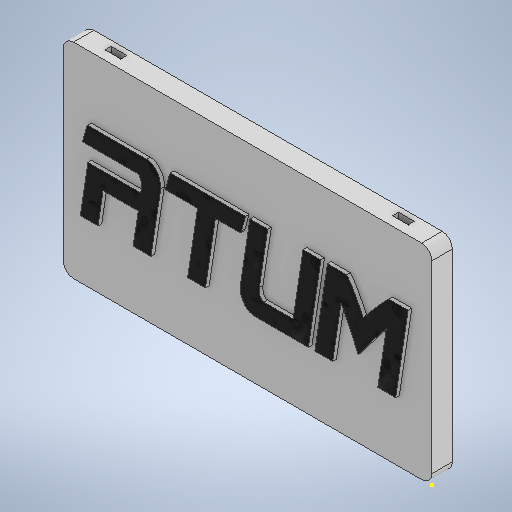
# Autodesk Inventor part: custom plate
Saved by Autodesk Inventor 2025.2 (Build 292293000, 293)
## iProperties
Created: 2024-12-05
Part Number: custom plate
Material: Generic
Document SubType Name: Modeling
Designer: Hunter Mathis
Density: 1 g/cm^3
Appearance: Default
Author: Hunter Mathis
Autodesk Inventor part; units mm, degrees
ref_plane "YZ Plane" through (0, 0, 0) normal (1, 0, 0) x (0, 1, 0)
ref_plane "XZ Plane" through (0, 0, 0) normal (0, 1, 0) x (-1, 0, 0)
ref_plane "XY Plane" through (0, 0, 0) normal (0, 0, 1) x (1, 0, 0)
sketch "Sketch1" plane through (0, 0, 0) normal (0, 0, 1) x (1, 0, 0)
  line L0 (0, 0) -> (-114.3, 0)
  line L1 (-114.3, 0) -> (-114.3, 63.5)
  line L2 (-114.3, 63.5) -> (0, 63.5)
  line L3 (0, 63.5) -> (0, 0)
  dimension "d7" = 114.3
  dimension "d8" = 63.5
  constraints: 8 end point, 2 parallel, 1 horizontal, 1 perpendicular
  measures "d7" distance of L1.end L2.end
  measures "d8" distance of L0.end L1.end
extrude "Extrusion1" add sketch "Sketch1" along normal blind 6.35
sketch "Sketch2" plane through (0, 0, 6.35) normal (0, 0, 1) x (1, 0, 0)
  line L0 (0, 0) -> (0, 63.5) projected
  line L1 (-114.3, 63.5) -> (-114.3, 0) projected
  line L2 (-114.3, 0) -> (0, 0) projected
  line L3 (0, 63.5) -> (-114.3, 63.5) projected
sketch "Sketch3" plane through (0, 0, 6.35) normal (0, 0, 1) x (1, 0, 0)
  line L0 (-110.6716, 35.2666) -> (-52.0005, 35.2666) construction
  line L1 (-52.0005, 35.2666) -> (-52.0005, 28.3217) construction
  line L2 (-52.0005, 28.3217) -> (-110.6716, 28.3217) construction
  line L3 (-110.6716, 28.3217) -> (-110.6716, 35.2666) construction
  line L4 (-114.3, 63.5) -> (-114.3, 0) projected
  line L5 (-107.8928, 19.0941) -> (-105.5257, 34.5523)
  line L6 (-105.5257, 34.5523) -> (-89.1412, 34.5523)
  line L7 (-89.1412, 34.5523) -> (-88.8942, 36.0343)
  spline S0 degree 2 poles (-88.8942, 36.0343) (-88.8119, 36.693) (-88.9766, 37.8663) (-89.3882, 38.7514) (-89.9852, 39.2659) (-90.3145, 39.2659) knots 0 0 0 1 2 3 4 4 4
  line L8 (-90.3145, 39.2659) -> (-107.1929, 39.2659)
  spline S1 degree 2 poles (-107.1929, 39.2659) (-106.9048, 40.3157) (-106.2667, 42.8063) (-105.9168, 43.8561) knots 0 0 0 1 2 2 2
  line L9 (-105.9168, 43.8561) -> (-105.6492, 44.4941)
  line L10 (-105.6492, 44.4941) -> (-87.3505, 44.4941)
  spline S2 degree 2 poles (-87.3505, 44.4941) (-86.6301, 44.4941) (-85.0451, 43.7737) (-83.7484, 42.3123) (-82.925, 40.1922) (-82.9662, 38.7308) knots 0 0 0 1 2 3 4 4 4
  line L11 (-82.9662, 38.7308) -> (-85.9714, 19.0941)
  line L12 (-85.9714, 19.0941) -> (-91.4878, 19.0941)
  line L13 (-91.4878, 19.0941) -> (-89.9234, 29.3241)
  line L14 (-89.9234, 29.3241) -> (-100.8121, 29.3241)
  line L15 (-100.8121, 29.3241) -> (-102.3764, 19.0941)
  line L16 (-102.3764, 19.0941) -> (-107.8928, 19.0941)
  spline S3 degree 2 poles (-81.5048, 39.2659) (-81.2166, 40.3157) (-80.5785, 42.8063) (-80.2492, 43.8561) knots 0 0 0 1 2 2 2
  line L17 (-80.2492, 43.8561) -> (-79.961, 44.4941)
  line L18 (-79.961, 44.4941) -> (-56.7017, 44.4941)
  spline S4 degree 2 poles (-56.7017, 44.4941) (-56.9693, 43.4444) (-57.628, 40.9538) (-57.9779, 39.904) knots 0 0 0 1 2 2 2
  line L19 (-57.9779, 39.904) -> (-58.2455, 39.2659)
  line L20 (-58.2455, 39.2659) -> (-66.0054, 39.2659)
  line L21 (-66.0054, 39.2659) -> (-69.0724, 19.0941)
  line L22 (-69.0724, 19.0941) -> (-74.5887, 19.0941)
  line L23 (-74.5887, 19.0941) -> (-71.5218, 39.2659)
  line L24 (-71.5218, 39.2659) -> (-81.5048, 39.2659)
  spline S5 degree 2 poles (-58.3072, 24.8575) (-58.369, 23.3961) (-57.525, 21.276) (-56.2283, 19.8146) (-54.6434, 19.0941) (-53.9435, 19.0941) knots 0 0 0 1 2 3 4 4 4
  line L25 (-53.9435, 19.0941) -> (-37.168, 19.0941)
  line L26 (-37.168, 19.0941) -> (-33.2983, 44.4941)
  line L27 (-33.2983, 44.4941) -> (-38.8147, 44.4941)
  line L28 (-38.8147, 44.4941) -> (-41.8816, 24.3223)
  line L29 (-41.8816, 24.3223) -> (-50.9795, 24.3223)
  spline S6 degree 2 poles (-50.9795, 24.3223) (-51.2882, 24.3223) (-51.8852, 24.8369) (-52.3174, 25.7014) (-52.4821, 26.8541) (-52.3792, 27.5334) knots 0 0 0 1 2 3 4 4 4
  line L30 (-52.3792, 27.5334) -> (-49.7857, 44.4941)
  line L31 (-49.7857, 44.4941) -> (-55.302, 44.4941)
  line L32 (-55.302, 44.4941) -> (-58.3072, 24.8575)
  line L33 (-31.2605, 44.4941) -> (-35.1508, 19.0941)
  line L34 (-35.1508, 19.0941) -> (-29.6344, 19.0941)
  line L35 (-29.6344, 19.0941) -> (-27.0409, 36.0755)
  spline S7 degree 2 poles (-27.0409, 36.0755) (-26.444, 35.0257) (-25.1472, 32.4116) (-23.8093, 29.5094) (-22.4302, 26.463) (-21.7716, 24.9604) knots 0 0 0 1 2 3 4 4 4
  line L36 (-21.7716, 24.9604) -> (-21.6892, 24.9604)
  spline S8 degree 2 poles (-21.6892, 24.9604) (-20.5777, 26.463) (-18.2518, 29.5505) (-16.0493, 32.4528) (-13.9498, 35.0257) (-13.0236, 36.0755) knots 0 0 0 1 2 3 4 4 4
  line L37 (-13.0236, 36.0755) -> (-15.6171, 19.0941)
  line L38 (-15.6171, 19.0941) -> (-10.1007, 19.0941)
  line L39 (-10.1007, 19.0941) -> (-6.231, 44.4941)
  line L40 (-6.231, 44.4941) -> (-12.2002, 44.4941)
  spline S9 degree 2 poles (-12.2002, 44.4941) (-13.6205, 43.2797) (-17.202, 39.1424) (-19.0545, 36.8783) knots 0 0 0 1 2 2 2
  line L41 (-19.0545, 36.8783) -> (-20.1249, 35.6021)
  spline S10 degree 2 poles (-20.1249, 35.6021) (-21.7716, 38.8543) (-24.221, 43.3209) (-25.2913, 44.4941) knots 0 0 0 1 2 2 2
  line L42 (-25.2913, 44.4941) -> (-31.2605, 44.4941)
  point P0 (0, 0)
  constraints: 2 other
extrude "Extrusion2" add sketch "Sketch3" along normal blind 1.143
fillet "Fillet2" radius 3.175 4 edges at (-114.3, 63.5, 3.175) (-114.3, 0, 3.175) (0, 0, 3.175) (0, 63.5, 3.175)
sketch "Sketch4" plane through (0, 0, 6.35) normal (0, 0, 1) x (1, 0, 0)
  point P0 (0, 0)
sketch "Sketch5" plane through (0, 0, 6.35) normal (0, 0, 1) x (1, 0, 0)
  point P0 (0, 0)
sketch "Sketch6" plane through (0, 0, 6.35) normal (0, 0, 1) x (1, 0, 0)
  point P0 (0, 0)
ref_plane "Work Plane1" through (-57.15, 3.175, 0) normal (1, 0, 0) x (0, 0, -1)
sketch "Sketch7" plane through (-111.125, 63.5, 0) normal (0, 1, 0) x (1, 0, 0)
  line L0 (107.95, -6.35) -> (0, -6.35) projected
  line L1 (107.95, 0) -> (0, 0) projected
  line L2 (0, -6.35) -> (0, -3.175)
  line L3 (0, -6.35) -> (0, 0) projected
  line L4 (0, 0) -> (0, -6.35) projected
  line L5 (0, -6.35) -> (0, -3.5306)
  line L6 (0, -3.5306) -> (6.985, -3.5306)
  line L7 (6.985, -3.5306) -> (11.8618, -3.5306)
  line L8 (11.8618, -3.5306) -> (11.8618, -1.651)
  line L9 (11.8618, -1.651) -> (6.985, -1.651)
  line L10 (6.985, -1.651) -> (6.985, -3.5306)
  point P0 (111.125, 0)
  dimension "d24" = 4.8768
  dimension "d25" = 1.8796
  dimension "d26" = 2.8194
  dimension "d27" = 6.985
  constraints: 14 end point, 2 horizontal, 2 parallel, 1 midpoint, 1 perpendicular, 1 point on line
  measures "d24" distance of L6.end L7.end
  measures "d25" distance of L7.end L8.end
  measures "d26" distance between parallel lines of L6 L0
  measures "d27" distance of L5.end L6.end
extrude "Extrusion3" cut sketch "Sketch7" against normal blind 9.652
sketch "Sketch8" plane through (-111.125, 0, 0) normal (0, -1, 0) x (1, 0, 0)
  line L0 (0, 0) -> (0, 6.35) projected
  line L1 (6.985, 3.5306) -> (6.985, 1.651) projected
  line L2 (11.8618, 1.651) -> (11.8618, 3.5306) projected
  line L3 (6.985, 1.651) -> (11.8618, 1.651)
  line L4 (11.8618, 1.651) -> (11.8618, 3.5306)
  line L5 (11.8618, 3.5306) -> (6.985, 3.5306)
  line L6 (6.985, 3.5306) -> (6.985, 1.651)
  line L7 (0, 0) -> (107.95, 0) projected
  point P0 (111.125, 0)
  constraints: 8 end point, 2 parallel, 1 horizontal, 1 perpendicular
extrude "Extrusion4" cut sketch "Sketch8" against normal blind 9.652
mirror "Mirror1" about plane through (-57.15, 3.175, 0) normal (1, 0, 0) of "Extrusion3"
mirror "Mirror2" about plane through (-57.15, 3.175, 0) normal (1, 0, 0) of "Extrusion4"
body "Solid1"
